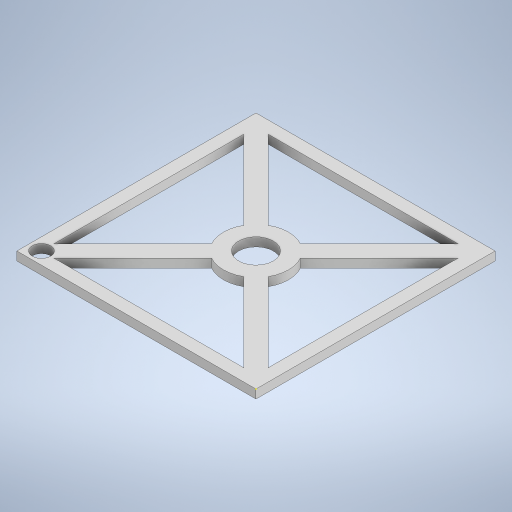
# Autodesk Inventor part: Pieza1
Saved by Autodesk Inventor 2023 (Build 270158000, 158)
## iProperties
Created: 2022-11-14
Part Number: Pieza1
Material: Genérico
Document SubType Name: Modeling
Designer: Jesus Tapia
Density: 1 g/cm^3
Appearance: Valor por defecto
Author: Jesus Tapia
Autodesk Inventor part; units mm, degrees
ref_plane "YZ Plane" through (0, 0, 0) normal (1, 0, 0) x (0, 1, 0)
ref_plane "XZ Plane" through (0, 0, 0) normal (0, 1, 0) x (-1, 0, 0)
ref_plane "XY Plane" through (0, 0, 0) normal (0, 0, 1) x (1, 0, 0)
sketch "Boceto4" plane through (0, 0, 0) normal (0, 1, 0) x (-1, 0, 0)
  line L0 (0, 0) -> (165, 0)
  line L1 (165, 0) -> (165, -165)
  line L2 (165, -165) -> (0, -165)
  line L3 (0, -165) -> (0, 0)
  dimension "d6" = 165
  dimension "d7" = 165
  constraints: 8 end point, 2 parallel, 1 horizontal, 1 perpendicular
  measures "d6" distance of L1.end L2.end
  measures "d7" distance of L0.end L1.end
extrude "Extrusión2" add sketch "Boceto4" along normal blind 6
sketch "Boceto5" plane through (0, 6, 0) normal (0, 1, 0) x (1, 0, 0)
  line L0 (-165, 0) -> (0, 0) projected
  line L1 (0, 165) -> (-165, 165) projected
  line L2 (0, 0) -> (-165, 165)
  line L3 (-165, 165) -> (0, 165)
  line L4 (-165, 165) -> (-165, 0) projected
  line L5 (0, 165) -> (-165, 0)
  circle A0 centre (-82.5, 82.5) radius 12
  circle A1 centre (-82.5, 82.5) radius 22.5
  line L6 (-82.5, 82.5) -> (-89.5711, 75.4289)
  line L7 (-82.5, 82.5) -> (-75.4289, 89.5711)
  line L8 (0, 0) -> (0, 165) projected
  line L9 (-82.5, 82.5) -> (-86.7426, 78.2574)
  line L10 (-86.7426, 78.2574) -> (-8.4853, 0)
  line L11 (-82.5, 82.5) -> (-78.2574, 86.7426)
  line L12 (-78.2574, 86.7426) -> (0, 8.4853)
  line L13 (-86.7426, 78.2574) -> (-165, 156.5147)
  line L14 (-78.2574, 86.7426) -> (-156.5147, 165)
  dimension "d10" = 24
  dimension "d11" = 45
  dimension "d14" = 6
  dimension "d15" = 6
  constraints: 22 end point, 8 point on line, 3 perpendicular, 2 centre point, 1 coincident, 1 collinear, 1 midpoint
  measures "d10" diameter of A0
  measures "d11" diameter of A1
  measures "d14" distance of L6.start L9.end
  measures "d15" distance of L6.start L11.end
extrude "Extrusión3" cut sketch "Boceto5" against normal through all contours A0 L13 L5 | L5 L10 A0 | L10 L5 L2 A0 | A0 L2 L5 L13 | L2 L5 L12 A0 | A0 L14 L5 L2 | L12 L5 A0 | A0 L5 L14
sketch "Boceto6" plane through (0, 6, 0) normal (0, 1, 0) x (1, 0, 0)
  line L0 (-165, 165) -> (-165, 0) projected
  line L1 (-165, 165) -> (0, 0)
  line L2 (0, 0) -> (0, 165) projected
  line L3 (-165, 0) -> (0, 165)
  circle A0 centre (-82.5, 82.5) radius 22.5
  line L4 (-82.5, 82.5) -> (-86.7426, 86.7426)
  line L5 (-86.7426, 86.7426) -> (-165, 8.4853)
  line L6 (-82.5, 82.5) -> (-78.2574, 78.2574)
  line L7 (-78.2574, 78.2574) -> (-156.5147, 0)
  line L8 (-165, 0) -> (0, 0) projected
  line L9 (-86.7426, 86.7426) -> (-8.4853, 165)
  line L10 (0, 165) -> (-165, 165) projected
  line L11 (-78.2574, 78.2574) -> (0, 156.5147)
  line L12 (-82.5, 82.5) -> (-78.2574, 86.7426)
  line L13 (-82.5, 82.5) -> (-78.2574, 86.7426)
  line L14 (-78.2574, 86.7426) -> (-156.5147, 165)
  line L15 (-82.5, 82.5) -> (-86.7426, 78.2574)
  line L16 (-86.7426, 78.2574) -> (-165, 156.5147)
  line L17 (-86.7426, 78.2574) -> (-8.4853, 0)
  line L18 (-165, 0) -> (-165, 165)
  line L19 (0, 165) -> (-165, 165)
  line L20 (0, 0) -> (0, 165)
  line L21 (-165, 0) -> (0, 0)
  line L22 (-165, 0) -> (0, 0) projected
  circle A1 centre (-82.5, 82.5) radius 12 projected
  line L23 (0, 165) -> (-165, 165) projected
  line L24 (-165, 165) -> (-165, 0) projected
  line L25 (-165, 0) -> (0, 0) projected
  line L26 (0, 0) -> (0, 165) projected
  circle A2 centre (-82.5, 82.5) radius 12 projected
  line L27 (0, 165) -> (-165, 165) projected
  line L28 (-165, 165) -> (-165, 0) projected
  line L29 (-165, 0) -> (0, 0) projected
  line L30 (0, 0) -> (0, 165) projected
  line L31 (0, -1.5147) -> (0, 8.4853)
  line L32 (0, 8.4853) -> (-165, 8.4853)
  line L33 (-156.5147, 0) -> (-156.5147, 165)
  line L34 (-8.4853, 0) -> (-8.4853, 165)
  line L35 (0, 156.5147) -> (-165, 156.5147)
  line L36 (-78.2574, 86.7426) -> (0, 8.4853)
  point P0 (-16.9706, 156.5147)
  point P1 (-148.0294, 156.5147)
  point P2 (-93.5911, 102.0764)
  point P3 (-71.4089, 102.0764)
  point P4 (-62.9236, 71.4089)
  point P5 (-8.4853, 16.9706)
  point P6 (-8.4853, 148.0294)
  point P7 (-62.9236, 93.5911)
  point P8 (-148.0294, 8.4853)
  point P9 (-16.9706, 8.4853)
  point P10 (-71.4089, 62.9236)
  point P11 (-93.5911, 62.9236)
  point P12 (-156.5147, 148.0294)
  point P13 (-156.5147, 16.9706)
  point P14 (-102.0764, 71.4089)
  point P15 (-102.0764, 93.5911)
  dimension "d18" = 45
  dimension "d19" = 6
  dimension "d20" = 6
  dimension "d21" = 6
  dimension "d22" = 6
  dimension "d24" = 10
  constraints: 48 end point, 13 point on line, 8 perpendicular, 2 collinear, 2 parallel, 1 centre point, 1 midpoint, 1 vertical
  measures "d18" diameter of A0
  measures "d19" distance of L4.start L4.end
  measures "d20" distance of L4.start L6.end
  measures "d21" distance of L4.start L12.end
  measures "d22" distance of L4.start L15.end
  measures "d24" distance of L31.start L31.end
extrude "Extrusión4" cut sketch "Boceto6" against normal through all contours L16 A0 L5 L33 | L35 L9 A0 L14 | L7 A0 L17 L32 | L34 L36 A0 L11
sketch "Boceto7" plane through (0, 6, 0) normal (0, 1, 0) x (1, 0, 0)
  point P0 (0, 0)
sketch "Boceto8" plane through (0, 6, 0) normal (0, 1, 0) x (1, 0, 0)
  line L0 (-148.0294, 156.5147) -> (-16.9706, 156.5147) projected
  line L1 (-165, 165) -> (-165, 0) projected
  line L2 (-16.9706, 8.4853) -> (-148.0294, 8.4853) projected
  line L3 (-16.9706, 156.5147) -> (-71.4089, 102.0764) projected
  circle A0 centre (-156.5147, 8.4853) radius 6.36
  point P0 (0, 0)
  constraints: 1 centre point
extrude "Extrusión5" cut sketch "Boceto8" against normal through all
